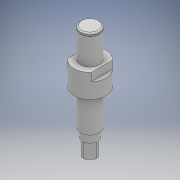
# Autodesk Inventor part: 3강
Saved by Autodesk Inventor 2018.3 (Build 223284000, 284)
## iProperties
Created: 2019-10-11
Part Number: 3강
Material: 일반
Document SubType Name: Modeling
Designer: MyTool
Density: 1 g/cm^3
Appearance: 기본값
Author: MyTool
Autodesk Inventor part; units mm, degrees
ref_plane "YZ Plane" through (0, 0, 0) normal (1, 0, 0) x (0, 1, 0)
ref_plane "XZ Plane" through (0, 0, 0) normal (0, 1, 0) x (-1, 0, 0)
ref_plane "XY Plane" through (0, 0, 0) normal (0, 0, 1) x (1, 0, 0)
sketch "스케치1" plane through (0, 0, 0) normal (1, 0, 0) x (0, 1, 0)
  line L0 (0, 0) -> (6.5, 0)
  line L1 (6.5, 0) -> (6.5, 20)
  line L2 (6.5, 20) -> (0, 20)
  line L3 (0, 20) -> (0, 0)
  line L4 (0, 20) -> (8, 20)
  line L5 (8, 20) -> (8, 50)
  line L6 (8, 50) -> (0, 50)
  line L7 (0, 50) -> (0, 20)
  line L8 (0, 50) -> (13.5, 50)
  line L9 (13.5, 50) -> (13.5, 70)
  line L10 (13.5, 70) -> (0, 70)
  line L11 (0, 70) -> (0, 50)
  line L12 (0, 70) -> (8, 70)
  line L13 (8, 70) -> (8, 95)
  line L14 (8, 95) -> (0, 95)
  line L15 (0, 95) -> (0, 70)
  dimension "d0" = 13
  dimension "d1" = 16
  dimension "d2" = 27
  dimension "d3" = 16
  dimension "d4" = 20
  dimension "d5" = 30
  dimension "d6" = 20
  dimension "d7" = 25
  constraints: 32 end point, 8 parallel, 4 horizontal, 4 perpendicular
  measures "d0" diameter of L1 L3
  measures "d1" diameter of L5 L7
  measures "d2" diameter of L9 L11
  measures "d3" diameter of L13 L15
  measures "d4" distance between parallel lines of L2 L0
  measures "d5" distance of L4.end L5.end
  measures "d6" distance between parallel lines of L10 L6
  measures "d7" distance between parallel lines of L14 L12
revolve "회전1" add sketch "스케치1" angle 360 about axis through (0, 0, 50) along (0, 0, -1)
sketch "스케치2" plane through (0, 0, 0) normal (0, 0, -1) x (-1, 0, 0)
  line L0 (0, 7.0711) -> (7.0711, 0)
  line L1 (7.0711, 0) -> (0, -7.0711)
  line L2 (0, -7.0711) -> (-7.0711, 0)
  line L3 (-7.0711, 0) -> (0, 7.0711)
  circle A0 centre (0, 0) radius 9.2868
  dimension "d9" = 10
  constraints: 8 end point, 2 coincident, 1 centre point, 9 other
  measures "d9" distance of L2.end L0.start
extrude "돌출1" cut sketch "스케치2" against normal blind 13
chamfer "모따기1" distance 1 angle 45 5 edges at (-0.2997, 6.4931, 0) (-6.5, 0, 0) (6.5, 0, 0) (0.2997, 6.4931, 0) (0, -6.5, 0)
sketch "스케치3" plane through (0, 0, 70) normal (0, 0, 1) x (1, 0, 0)
  circle A0 centre (0, 0) radius 13.5 projected
  line L0 (-10.0623, 9) -> (-10.0623, -9)
  line L1 (-10.0623, 9) -> (-13.5, 9)
  line L2 (-13.5, 9) -> (-13.5, -9)
  line L3 (-13.5, -9) -> (-10.0623, -9)
  dimension "d15" = 18
  constraints: 8 end point, 2 perpendicular, 2 point on circle, 1 horizontal, 1 vertical
  measures "d15" distance of L0.start L0.end
extrude "돌출2" cut sketch "스케치3" against normal blind 7 contours L0 A0 | A0 L2 L1 | L3 L2 A0 picked at (-11.0757, -1.0838)
mirror "미러1" about plane through (0, 0, 0) normal (1, 0, 0) of "돌출2"
sketch "스케치4" plane through (0, 0, 0) normal (1, 0, 0) x (0, 1, 0)
  line L0 (8, 92.35) -> (7.6, 92.35)
  line L1 (7.6, 92.35) -> (7.6, 93.5)
  line L2 (7.6, 93.5) -> (8, 93.5)
  line L3 (8, 93.5) -> (8, 92.35)
  line L4 (8, 95) -> (8, 70) projected
  line L5 (0, -19) -> (0, 114) projected
  point P0 (0, 0)
  dimension "d19" = 1.15
  dimension "d20" = 1.5
  dimension "d21" = 0.4
  constraints: 8 end point, 2 parallel, 1 collinear, 1 horizontal, 1 perpendicular
  measures "d19" distance of L2.end L0.start
  measures "d20" distance from line of L4.start L2
  measures "d21" distance of L1.end L2.end
revolve "회전2" cut sketch "스케치4" angle 360 about axis through (0, 0, -10) along (0, 0, 1)
chamfer "모따기2" distance 1 angle 45 1 edges at (0, -8, 95)
